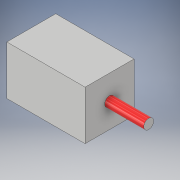
# Autodesk Inventor part: BaneBot220GearBox
Saved by Autodesk Inventor 2018.2 (Build 222227000, 227)
## iProperties
Created: 2018-02-07
Part Number: BaneBot220GearBox
Material: Generic
Document SubType Name: Modeling
Designer: steele
Density: 1 g/cm^3
Appearance: Default
Author: steele
Autodesk Inventor part; units mm, degrees
ref_plane "YZ Plane" through (0, 0, 0) normal (1, 0, 0) x (0, 1, 0)
ref_plane "XZ Plane" through (0, 0, 0) normal (0, 1, 0) x (-1, 0, 0)
ref_plane "XY Plane" through (0, 0, 0) normal (0, 0, 1) x (1, 0, 0)
sketch "Sketch1" plane through (0, 0, 0) normal (0, 1, 0) x (-1, 0, 0)
  line L0 (50.8, 31.75) -> (-50.8, 31.75)
  line L1 (-50.8, 31.75) -> (-50.8, -31.75)
  line L2 (-50.8, -31.75) -> (50.8, -31.75)
  line L3 (50.8, -31.75) -> (50.8, 31.75)
  line L4 (50.8, 31.75) -> (-50.8, -31.75) construction
  line L5 (-50.8, 31.75) -> (50.8, -31.75) construction
  point P0 (0, 0)
  dimension "d0" = 101.6
  dimension "d1" = 63.5
  constraints: 12 end point, 2 midpoint, 2 parallel, 1 horizontal, 1 perpendicular
  measures "d0" distance of L1.end L2.end
  measures "d1" distance of L2.end L0.start
extrude "Extrusion1" add sketch "Sketch1" along normal blind 63.5
sketch "Sketch2" plane through (0, 0, 0) normal (0, -1, 0) x (1, 0, 0)
  line L0 (17.272, 12.7) -> (-17.272, 12.7) construction
  line L1 (-17.272, 12.7) -> (-17.272, -12.7) construction
  line L2 (-17.272, -12.7) -> (17.272, -12.7) construction
  line L3 (17.272, -12.7) -> (17.272, 12.7) construction
  line L4 (17.272, 12.7) -> (-17.272, -12.7) construction
  line L5 (-17.272, 12.7) -> (17.272, -12.7) construction
  point P0 (0, 0)
  dimension "d5" = 34.544
  dimension "d6" = 25.4
  constraints: 12 end point, 4 coincident, 2 midpoint, 2 parallel, 1 horizontal, 1 perpendicular
  measures "d5" distance of L0.start L0.end
  measures "d6" distance of L1.end L0.end
hole "Hole1" at (17.272, 0, -12.7) at (-17.272, 0, -12.7) at (-17.272, 0, 12.7) at (17.272, 0, 12.7) direction (0, 1, 0) diameter 3.9624 depth 12.7 tip angle 118 thread size "10-32 UNF" class "2B" standard "ANSI Unified Screw Threads"
sketch "Sketch3" plane through (50.8, 0, 31.75) normal (1, 0, 0) x (0, 0, -1)
  circle A0 centre (31.75, 31.75) radius 6.35
  line L0 (0, 0) -> (0, 63.5) projected
  line L1 (0, 0) -> (63.5, 0) projected
  point P0 (31.75, 0)
  dimension "d14" = 12.7
  dimension "d15" = 31.75
  dimension "d16" = 31.75
  constraints: 1 centre point
  measures "d14" diameter of A0
  measures "d15" distance from line of A0.centre L0
  measures "d16" distance from line of A0.centre L1
extrude "Extrusion2" add sketch "Sketch3" along normal blind 50.8
body "Solid1"
